Autodesk Inventor part; units mm, degrees
note: some values were not read from the file. Chosen so that the rebuilt part matches the saved one: arc direction of "Выдавливание3".
(part 2 of 2)
  line L336 (-0.5075, 4.2102) -> (-0.3994, 4.0495) projected
  line L337 (-0.6209, 4.363) -> (-0.5075, 4.2102) projected
  line L338 (-0.7397, 4.5072) -> (-0.6209, 4.363) projected
  line L339 (-0.8641, 4.6418) -> (-0.7397, 4.5072) projected
  line L340 (-0.9947, 4.7654) -> (-0.8641, 4.6418) projected
  line L341 (-1.1329, 4.8749) -> (-0.9947, 4.7654) projected
  line L342 (-1.2046, 4.9247) -> (-1.1329, 4.8749) projected
  line L343 (-1.2728, 4.9814) -> (-1.2046, 4.9247) projected
  line L344 (-1.3354, 5.0493) -> (-1.2728, 4.9814) projected
  line L345 (-1.3631, 5.0902) -> (-1.3354, 5.0493) projected
  line L346 (-1.3863, 5.1406) -> (-1.3631, 5.0902) projected
  line L347 (-1.3841, 5.2433) -> (-1.3863, 5.1406) projected
  line L348 (-1.0111, 6.1437) -> (-1.3841, 5.2433) projected
  line L349 (-0.9401, 6.2178) -> (-1.0111, 6.1437) projected
  line L350 (-0.8881, 6.2371) -> (-0.9401, 6.2178) projected
  line L351 (-0.8395, 6.2464) -> (-0.8881, 6.2371) projected
  line L352 (-0.7473, 6.2501) -> (-0.8395, 6.2464) projected
  line L353 (-0.659, 6.242) -> (-0.7473, 6.2501) projected
  line L354 (-0.573, 6.2266) -> (-0.659, 6.242) projected
  line L355 (-0.3979, 6.2063) -> (-0.573, 6.2266) projected
  line L356 (-0.2181, 6.2013) -> (-0.3979, 6.2063) projected
  line L357 (-0.035, 6.2085) -> (-0.2181, 6.2013) projected
  line L358 (0.151, 6.2264) -> (-0.035, 6.2085) projected
  line L359 (0.3392, 6.2543) -> (0.151, 6.2264) projected
  line L360 (0.5293, 6.2915) -> (0.3392, 6.2543) projected
  line L361 (0.721, 6.3378) -> (0.5293, 6.2915) projected
  line L362 (0.8657, 6.3782) -> (0.721, 6.3378) projected
  line L363 (1.0789, 7.4504) -> (0.8657, 6.3782) projected
  line L364 (0.9608, 7.543) -> (1.0789, 7.4504) projected
  line L365 (0.8013, 7.6591) -> (0.9608, 7.543) projected
  line L366 (0.6399, 7.7662) -> (0.8013, 7.6591) projected
  line L367 (0.4767, 7.864) -> (0.6399, 7.7662) projected
  line L368 (0.3118, 7.9518) -> (0.4767, 7.864) projected
  line L369 (0.1453, 8.0285) -> (0.3118, 7.9518) projected
  line L370 (-0.0227, 8.0927) -> (0.1453, 8.0285) projected
  line L371 (-0.1922, 8.141) -> (-0.0227, 8.0927) projected
  line L372 (-0.2775, 8.1596) -> (-0.1922, 8.141) projected
  line L373 (-0.3622, 8.1859) -> (-0.2775, 8.1596) projected
  line L374 (-0.446, 8.2246) -> (-0.3622, 8.1859) projected
  line L375 (-0.4873, 8.2518) -> (-0.446, 8.2246) projected
  line L376 (-0.528, 8.2895) -> (-0.4873, 8.2518) projected
  line L377 (-0.5652, 8.3852) -> (-0.528, 8.2895) projected
  line L378 (-0.5652, 9.3598) -> (-0.5652, 8.3852) projected
  line L379 (-0.528, 9.4555) -> (-0.5652, 9.3598) projected
  line L380 (-0.4873, 9.4932) -> (-0.528, 9.4555) projected
  line L381 (-0.446, 9.5204) -> (-0.4873, 9.4932) projected
  line L382 (-0.3622, 9.5591) -> (-0.446, 9.5204) projected
  line L383 (-0.2775, 9.5854) -> (-0.3622, 9.5591) projected
  line L384 (-0.1922, 9.604) -> (-0.2775, 9.5854) projected
  line L385 (-0.0227, 9.6523) -> (-0.1922, 9.604) projected
  line L386 (0.1453, 9.7165) -> (-0.0227, 9.6523) projected
  line L387 (0.3118, 9.7933) -> (0.1453, 9.7165) projected
  line L388 (0.4767, 9.881) -> (0.3118, 9.7933) projected
  line L389 (0.6399, 9.9788) -> (0.4767, 9.881) projected
  line L390 (0.8013, 10.0859) -> (0.6399, 9.9788) projected
  line L391 (0.9608, 10.202) -> (0.8013, 10.0859) projected
  line L392 (1.0789, 10.2947) -> (0.9608, 10.202) projected
  line L393 (0.8657, 11.3669) -> (1.0789, 10.2947) projected
  line L394 (0.721, 11.4073) -> (0.8657, 11.3669) projected
  line L395 (0.5293, 11.4535) -> (0.721, 11.4073) projected
  line L396 (0.3392, 11.4907) -> (0.5293, 11.4535) projected
  line L397 (0.151, 11.5186) -> (0.3392, 11.4907) projected
  line L398 (-0.035, 11.5365) -> (0.151, 11.5186) projected
  line L399 (-0.2181, 11.5437) -> (-0.035, 11.5365) projected
  line L400 (-0.3979, 11.5388) -> (-0.2181, 11.5437) projected
  line L401 (-0.573, 11.5185) -> (-0.3979, 11.5388) projected
  line L402 (-0.659, 11.5031) -> (-0.573, 11.5185) projected
  line L403 (-0.7473, 11.4949) -> (-0.659, 11.5031) projected
  line L404 (-0.8395, 11.4986) -> (-0.7473, 11.4949) projected
  line L405 (-0.8881, 11.5079) -> (-0.8395, 11.4986) projected
  line L406 (-0.9401, 11.5272) -> (-0.8881, 11.5079) projected
  line L407 (-1.0111, 11.6014) -> (-0.9401, 11.5272) projected
  line L408 (-1.3841, 12.5018) -> (-1.0111, 11.6014) projected
  line L409 (-1.3863, 12.6044) -> (-1.3841, 12.5018) projected
  line L410 (-1.3631, 12.6548) -> (-1.3863, 12.6044) projected
  line L411 (-1.3354, 12.6958) -> (-1.3631, 12.6548) projected
  line L412 (-1.2728, 12.7636) -> (-1.3354, 12.6958) projected
  line L413 (-1.2046, 12.8203) -> (-1.2728, 12.7636) projected
  line L414 (-1.1329, 12.8702) -> (-1.2046, 12.8203) projected
  line L415 (-0.9947, 12.9796) -> (-1.1329, 12.8702) projected
  line L416 (-0.8641, 13.1032) -> (-0.9947, 12.9796) projected
  line L417 (-0.7397, 13.2378) -> (-0.8641, 13.1032) projected
  line L418 (-0.6209, 13.382) -> (-0.7397, 13.2378) projected
  line L419 (-0.5075, 13.5348) -> (-0.6209, 13.382) projected
  line L420 (-0.3994, 13.6956) -> (-0.5075, 13.5348) projected
  line L421 (-0.2965, 13.8638) -> (-0.3994, 13.6956) projected
  line L422 (-0.2228, 13.9947) -> (-0.2965, 13.8638) projected
  line L423 (-0.8302, 14.9036) -> (-0.2228, 13.9947) projected
  line L424 (-0.9793, 14.8856) -> (-0.8302, 14.9036) projected
  line L425 (-1.1741, 14.8549) -> (-0.9793, 14.8856) projected
  line L426 (-1.364, 14.8166) -> (-1.1741, 14.8549) projected
  line L427 (-1.5485, 14.7703) -> (-1.364, 14.8166) projected
  line L428 (-1.7272, 14.7157) -> (-1.5485, 14.7703) projected
  line L429 (-1.8991, 14.6523) -> (-1.7272, 14.7157) projected
  line L430 (-2.0633, 14.5789) -> (-1.8991, 14.6523) projected
  line L431 (-2.2174, 14.4931) -> (-2.0633, 14.5789) projected
  line L432 (-2.2909, 14.446) -> (-2.2174, 14.4931) projected
  line L433 (-2.3693, 14.4047) -> (-2.2909, 14.446) projected
  line L434 (-2.4559, 14.3728) -> (-2.3693, 14.4047) projected
  line L435 (-2.5044, 14.3628) -> (-2.4559, 14.3728) projected
  line L436 (-2.5599, 14.3607) -> (-2.5044, 14.3628) projected
  line L437 (-2.6538, 14.4021) -> (-2.5599, 14.3607) projected
  line L438 (-3.3429, 15.0912) -> (-2.6538, 14.4021) projected
  line L439 (-3.3843, 15.1852) -> (-3.3429, 15.0912) projected
  line L440 (-3.3822, 15.2406) -> (-3.3843, 15.1852) projected
  line L441 (-3.3722, 15.2891) -> (-3.3822, 15.2406) projected
  line L442 (-3.3403, 15.3757) -> (-3.3722, 15.2891) projected
  line L443 (-3.299, 15.4541) -> (-3.3403, 15.3757) projected
  line L444 (-3.2519, 15.5277) -> (-3.299, 15.4541) projected
  line L445 (-3.1661, 15.6817) -> (-3.2519, 15.5277) projected
  line L446 (-3.0927, 15.8459) -> (-3.1661, 15.6817) projected
  line L447 (-3.0293, 16.0179) -> (-3.0927, 15.8459) projected
  line L448 (-2.9747, 16.1965) -> (-3.0293, 16.0179) projected
  line L449 (-2.9285, 16.381) -> (-2.9747, 16.1965) projected
  line L450 (-2.8901, 16.5709) -> (-2.9285, 16.381) projected
  line L451 (-2.8594, 16.7658) -> (-2.8901, 16.5709) projected
  line L452 (-2.8414, 16.9149) -> (-2.8594, 16.7658) projected
  line L453 (-3.7504, 17.5222) -> (-2.8414, 16.9149) projected
  line L454 (-3.8812, 17.4485) -> (-3.7504, 17.5222) projected
  line L455 (-4.0495, 17.3456) -> (-3.8812, 17.4485) projected
  line L456 (-4.2102, 17.2375) -> (-4.0495, 17.3456) projected
  line L457 (-4.363, 17.1241) -> (-4.2102, 17.2375) projected
  line L458 (-4.5072, 17.0053) -> (-4.363, 17.1241) projected
  line L459 (-4.6418, 16.8809) -> (-4.5072, 17.0053) projected
  line L460 (-4.7654, 16.7503) -> (-4.6418, 16.8809) projected
  line L461 (-4.8749, 16.6121) -> (-4.7654, 16.7503) projected
  line L462 (-4.9247, 16.5404) -> (-4.8749, 16.6121) projected
  line L463 (-4.9814, 16.4722) -> (-4.9247, 16.5404) projected
  line L464 (-5.0493, 16.4097) -> (-4.9814, 16.4722) projected
  line L465 (-5.0902, 16.3819) -> (-5.0493, 16.4097) projected
  line L466 (-5.1406, 16.3587) -> (-5.0902, 16.3819) projected
  line L467 (-5.2433, 16.3609) -> (-5.1406, 16.3587) projected
  line L468 (-6.1437, 16.7339) -> (-5.2433, 16.3609) projected
  line L469 (-6.2178, 16.8049) -> (-6.1437, 16.7339) projected
  line L470 (-6.2371, 16.8569) -> (-6.2178, 16.8049) projected
  line L471 (-6.2464, 16.9055) -> (-6.2371, 16.8569) projected
  line L472 (-6.2501, 16.9977) -> (-6.2464, 16.9055) projected
  line L473 (-6.242, 17.086) -> (-6.2501, 16.9977) projected
  line L474 (-6.2266, 17.172) -> (-6.242, 17.086) projected
  line L475 (-6.2063, 17.3471) -> (-6.2266, 17.172) projected
  line L476 (-6.2013, 17.5269) -> (-6.2063, 17.3471) projected
  line L477 (-6.2085, 17.71) -> (-6.2013, 17.5269) projected
  line L478 (-6.2264, 17.896) -> (-6.2085, 17.71) projected
  line L479 (-6.2543, 18.0842) -> (-6.2264, 17.896) projected
  line L480 (-6.2915, 18.2743) -> (-6.2543, 18.0842) projected
  line L481 (-6.3378, 18.466) -> (-6.2915, 18.2743) projected
  line L482 (-6.3782, 18.6107) -> (-6.3378, 18.466) projected
  line L483 (-7.4504, 18.824) -> (-6.3782, 18.6107) projected
  line L484 (-7.543, 18.7058) -> (-7.4504, 18.824) projected
  line L485 (-7.6591, 18.5463) -> (-7.543, 18.7058) projected
  line L486 (-7.7662, 18.3849) -> (-7.6591, 18.5463) projected
  line L487 (-7.864, 18.2217) -> (-7.7662, 18.3849) projected
  line L488 (-7.9518, 18.0568) -> (-7.864, 18.2217) projected
  line L489 (-8.0285, 17.8903) -> (-7.9518, 18.0568) projected
  line L490 (-8.0927, 17.7224) -> (-8.0285, 17.8903) projected
  line L491 (-8.141, 17.5528) -> (-8.0927, 17.7224) projected
  line L492 (-8.1596, 17.4675) -> (-8.141, 17.5528) projected
  line L493 (-8.1859, 17.3828) -> (-8.1596, 17.4675) projected
  line L494 (-8.2246, 17.299) -> (-8.1859, 17.3828) projected
  line L495 (-8.2518, 17.2577) -> (-8.2246, 17.299) projected
  line L496 (-8.2895, 17.217) -> (-8.2518, 17.2577) projected
  line L497 (-8.3852, 17.1798) -> (-8.2895, 17.217) projected
  line L498 (-9.3598, 17.1798) -> (-8.3852, 17.1798) projected
  line L499 (-9.4555, 17.217) -> (-9.3598, 17.1798) projected
  line L500 (-9.4932, 17.2577) -> (-9.4555, 17.217) projected
  line L501 (-9.5204, 17.299) -> (-9.4932, 17.2577) projected
  line L502 (-9.5591, 17.3828) -> (-9.5204, 17.299) projected
  line L503 (-9.5854, 17.4675) -> (-9.5591, 17.3828) projected
  line L504 (-9.604, 17.5528) -> (-9.5854, 17.4675) projected
  line L505 (-9.6523, 17.7224) -> (-9.604, 17.5528) projected
  line L506 (-9.7165, 17.8903) -> (-9.6523, 17.7224) projected
  line L507 (-9.7933, 18.0568) -> (-9.7165, 17.8903) projected
  line L508 (-9.881, 18.2217) -> (-9.7933, 18.0568) projected
  line L509 (-9.9788, 18.3849) -> (-9.881, 18.2217) projected
  line L510 (-10.0859, 18.5463) -> (-9.9788, 18.3849) projected
  line L511 (-10.202, 18.7058) -> (-10.0859, 18.5463) projected
  line L512 (-10.2947, 18.824) -> (-10.202, 18.7058) projected
  line L513 (-11.3669, 18.6107) -> (-10.2947, 18.824) projected
  line L514 (-11.4073, 18.466) -> (-11.3669, 18.6107) projected
  line L515 (-11.4535, 18.2743) -> (-11.4073, 18.466) projected
  line L516 (-11.4907, 18.0842) -> (-11.4535, 18.2743) projected
  line L517 (-7.0717, 6.8191) -> (-7.3688, 6.5926) projected
  line L518 (-6.8084, 7.084) -> (-7.0717, 6.8191) projected
  line L519 (-6.5837, 7.3824) -> (-6.8084, 7.084) projected
  line L520 (-6.4017, 7.7087) -> (-6.5837, 7.3824) projected
  line L521 (-5.6712, 8.4057) -> (-6.4017, 7.7087) projected
  line L522 (-2.7091, 8.995) -> (-5.6712, 8.4057) projected
  line L523 (-2.1823, 8.548) -> (-2.7091, 8.995) projected
  line L524 (-2.2189, 8.1017) -> (-2.1823, 8.548) projected
  line L525 (-2.2853, 7.6589) -> (-2.2189, 8.1017) projected
  line L526 (-2.3811, 7.2214) -> (-2.2853, 7.6589) projected
  line L527 (-2.5059, 6.7914) -> (-2.3811, 7.2214) projected
  line L528 (-2.6592, 6.3707) -> (-2.5059, 6.7914) projected
  line L529 (-2.8403, 5.9611) -> (-2.6592, 6.3707) projected
  line L530 (-3.0483, 5.5646) -> (-2.8403, 5.9611) projected
  line L531 (-3.2823, 5.1828) -> (-3.0483, 5.5646) projected
  line L532 (-3.5413, 4.8176) -> (-3.2823, 5.1828) projected
  line L533 (-3.8242, 4.4704) -> (-3.5413, 4.8176) projected
  line L534 (-4.1296, 4.143) -> (-3.8242, 4.4704) projected
  line L535 (-4.4562, 3.8366) -> (-4.1296, 4.143) projected
  line L536 (-4.8025, 3.5528) -> (-4.4562, 3.8366) projected
  line L537 (-5.167, 3.2928) -> (-4.8025, 3.5528) projected
  line L538 (-5.5481, 3.0576) -> (-5.167, 3.2928) projected
  line L539 (-5.9441, 2.8485) -> (-5.5481, 3.0576) projected
  line L540 (-6.3531, 2.6663) -> (-5.9441, 2.8485) projected
  line L541 (-6.7734, 2.5119) -> (-6.3531, 2.6663) projected
  line L542 (-7.2031, 2.3858) -> (-6.7734, 2.5119) projected
  line L543 (-7.6402, 2.2888) -> (-7.2031, 2.3858) projected
  line L544 (-8.0829, 2.2211) -> (-7.6402, 2.2888) projected
  line L545 (-8.5291, 2.1833) -> (-8.0829, 2.2211) projected
  line L546 (-8.9768, 2.1752) -> (-8.5291, 2.1833) projected
  line L547 (-9.424, 2.1972) -> (-8.9768, 2.1752) projected
  line L548 (-9.7984, 2.7778) -> (-9.424, 2.1972) projected
  line L549 (-8.8276, 5.6377) -> (-9.7984, 2.7778) projected
  line L550 (-8.0411, 6.271) -> (-8.8276, 5.6377) projected
  line L551 (-7.6939, 6.4087) -> (-8.0411, 6.271) projected
  line L552 (-7.3688, 6.5926) -> (-7.6939, 6.4087) projected
  line L553 (-13.2172, 3.7746) -> (-12.8668, 3.4958) projected
  line L554 (-13.5481, 4.0763) -> (-13.2172, 3.7746) projected
  line L555 (-13.8581, 4.3994) -> (-13.5481, 4.0763) projected
  line L556 (-14.1458, 4.7425) -> (-13.8581, 4.3994) projected
  line L557 (-14.41, 5.1041) -> (-14.1458, 4.7425) projected
  line L558 (-14.6494, 5.4825) -> (-14.41, 5.1041) projected
  line L559 (-14.863, 5.8761) -> (-14.6494, 5.4825) projected
  line L560 (-15.0498, 6.283) -> (-14.863, 5.8761) projected
  line L561 (-15.209, 6.7015) -> (-15.0498, 6.283) projected
  line L562 (-15.3399, 7.1298) -> (-15.209, 6.7015) projected
  line L563 (-15.4419, 7.5658) -> (-15.3399, 7.1298) projected
  line L564 (-15.5145, 8.0076) -> (-15.4419, 7.5658) projected
  line L565 (-15.5574, 8.4533) -> (-15.5145, 8.0076) projected
  line L566 (-15.5705, 8.9009) -> (-15.5574, 8.4533) projected
  line L567 (-15.5537, 9.3484) -> (-15.5705, 8.9009) projected
  line L568 (-15.5069, 9.7937) -> (-15.5537, 9.3484) projected
  line L569 (-15.4305, 10.235) -> (-15.5069, 9.7937) projected
  line L570 (-15.3249, 10.6701) -> (-15.4305, 10.235) projected
  line L571 (-15.1903, 11.0972) -> (-15.3249, 10.6701) projected
  line L572 (-15.0276, 11.5143) -> (-15.1903, 11.0972) projected
  line L573 (-14.8373, 11.9197) -> (-15.0276, 11.5143) projected
  line L574 (-14.6204, 12.3114) -> (-14.8373, 11.9197) projected
  line L575 (-14.3778, 12.6878) -> (-14.6204, 12.3114) projected
  line L576 (-13.6877, 12.7217) -> (-14.3778, 12.6878) projected
  line L577 (-11.6964, 10.451) -> (-13.6877, 12.7217) projected
  line L578 (-11.5412, 9.4533) -> (-11.6964, 10.451) projected
  line L579 (-11.5955, 9.0837) -> (-11.5412, 9.4533) projected
  line L580 (-11.5988, 8.7102) -> (-11.5955, 9.0837) projected
  line L581 (-11.5512, 8.3397) -> (-11.5988, 8.7102) projected
  line L582 (-11.4534, 7.9792) -> (-11.5512, 8.3397) projected
  line L583 (-11.3074, 7.6353) -> (-11.4534, 7.9792) projected
  line L584 (-11.1158, 7.3147) -> (-11.3074, 7.6353) projected
  line L585 (-10.8774, 6.3335) -> (-11.1158, 7.3147) projected
  line L586 (-11.8482, 3.4736) -> (-10.8774, 6.3335) projected
  line L587 (-12.4987, 3.2409) -> (-11.8482, 3.4736) projected
  line L588 (-12.8668, 3.4958) -> (-12.4987, 3.2409) projected
  circle A2 centre (-8.8725, 8.8725) radius 2.7311
  point P0 (0, 0)
  point P1 (-11.2279, 9.3851)
  point P2 (-11.3073, 7.6353)
  point P3 (-8.0411, 6.271)
  point P4 (-6.4018, 7.7086)
  point P5 (-7.0352, 10.8933)
  point P6 (-7.3282, 11.1251)
  point P7 (-8.7264, 11.5997)
  point P8 (-11.3074, 7.6354)
  point P9 (-7.0719, 6.819)
  point P10 (-7.0716, 6.8192)
  point P11 (-7.3281, 11.125)
  point P12 (-6.5836, 7.3825)
  point P13 (-6.5837, 7.3823)
  point P14 (-6.8083, 7.0841)
  point P15 (-6.8084, 7.084)
  point P16 (-7.3687, 6.5926)
  point P17 (-7.3688, 6.5926)
  point P18 (-7.6939, 6.4088)
  point P19 (-7.694, 6.4087)
  point P20 (-11.5512, 8.3396)
  point P21 (-11.5512, 8.3397)
  point P22 (-8.7265, 11.5998)
  point P23 (-11.1158, 7.3147)
  point P24 (-11.5412, 9.4533)
  constraints: 1 coincident, 3 other
extrude "Выдавливание3" add sketch "Эскиз3" along normal blind 4 contours A1 L36 A0 L35 L34 L33 A2 L520 L519 L518 L517 L552 L551 L584 L583 L582 L581 L580 L579 L2 L1 L0 | L2 A2 | A2 L33 | L580 A2 | A2 L520 | L584 A2 | A2 L552 | L551 A2
